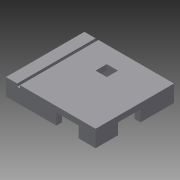
# Autodesk Inventor part: Casing Top
Saved by Autodesk Inventor 2014 SP1 (Build 180222100, 222)
## iProperties
Created: 2013-10-01
Part Number: Casing Top
Material: Generic
Document SubType Name: Modeling
Designer: Anthony
Density: 1 g/cm^3
Appearance: Default
Author: Anthony
Autodesk Inventor part; units mm, degrees
ref_plane "YZ Plane" through (0, 0, 0) normal (1, 0, 0) x (0, 1, 0)
ref_plane "XZ Plane" through (0, 0, 0) normal (0, 1, 0) x (-1, 0, 0)
ref_plane "XY Plane" through (0, 0, 0) normal (0, 0, 1) x (1, 0, 0)
sketch "Sketch1" plane through (0, 0, 0) normal (0, 1, 0) x (-1, 0, 0)
  line L0 (0, 0) -> (-50.8, 0)
  line L1 (-50.8, 0) -> (-50.8, 44.45)
  line L2 (-50.8, 44.45) -> (0, 44.45)
  line L3 (0, 44.45) -> (0, 0)
  dimension "d0" = 50.8
  dimension "d1" = 44.45
  constraints: 8 end point, 2 parallel, 1 horizontal, 1 perpendicular
  measures "d0" distance of L1.end L2.end
  measures "d1" distance of L0.end L1.end
extrude "Extrusion1" add sketch "Sketch1" along normal blind 3.175
sketch "Sketch2" plane through (0, 0, 44.45) normal (0, -1, 0) x (1, 0, 0)
  line L0 (50.8, 0) -> (0, 0)
  line L1 (0, 0) -> (0, -44.45)
  line L2 (0, -44.45) -> (50.8, -44.45)
  line L3 (50.8, -44.45) -> (50.8, 0)
  line L4 (3.175, -3.175) -> (47.625, -3.175)
  line L5 (47.625, -3.175) -> (47.625, -41.275)
  line L6 (47.625, -41.275) -> (3.175, -41.275)
  line L7 (3.175, -41.275) -> (3.175, -3.175)
  dimension "d4" = 3.175
  dimension "d7" = 3.175
  dimension "d5" = 3.175
  dimension "d6" = 3.175
  constraints: 16 end point, 2 parallel, 1 horizontal, 1 perpendicular
  measures "d4" distance between parallel lines of L1 L7
  measures "d7" distance between parallel lines of L0 L4
  measures "d5" distance between parallel lines of L2 L6
  measures "d6" distance between parallel lines of L3 L5
extrude "Extrusion2" add sketch "Sketch2" along normal blind 6.35
sketch "Sketch3" plane through (0, -6.35, 44.45) normal (0, 0, 1) x (1, 0, 0)
  line L0 (28.575, 0) -> (41.275, 0)
  line L1 (41.275, 0) -> (41.275, 6.35)
  line L2 (41.275, 6.35) -> (28.575, 6.35)
  line L3 (28.575, 6.35) -> (28.575, 0)
  line L4 (50.8, 0) -> (0, 0) projected
  line L5 (0, 9.525) -> (50.8, 9.525) projected
  line L6 (0, 9.525) -> (0, 0) projected
  dimension "d18" = 0
  dimension "d20" = 28.575
  dimension "d21" = 41.275
  dimension "d27" = 6.35
  constraints: 8 end point, 2 parallel, 1 horizontal, 1 perpendicular
  measures "d18" distance between parallel lines of L0 L4
  measures "d20" distance between parallel lines of L3 L6
  measures "d21" distance between parallel lines of L6 L1
  measures "d27" distance of L0.end L1.end
extrude "Extrusion3" cut sketch "Sketch3" against normal blind 3.175
sketch "Sketch4" plane through (50.8, 3.175, 44.45) normal (1, 0, 0) x (0, 0, -1)
  line L0 (0, 0) -> (0, -9.525) projected
  line L1 (44.45, -9.525) -> (0, -9.525) projected
  line L2 (12.7, -9.525) -> (25.4, -9.525)
  line L3 (25.4, -9.525) -> (25.4, -3.175)
  line L4 (25.4, -3.175) -> (12.7, -3.175)
  line L5 (12.7, -3.175) -> (12.7, -9.525)
  point P0 (44.45, -3.175)
  dimension "d22" = 6.35
  dimension "d23" = 12.7
  dimension "d24" = 25.4
  constraints: 8 end point, 2 parallel, 1 horizontal, 1 perpendicular, 1 point on line
  measures "d22" distance of L4.end L2.start
  measures "d23" distance between parallel lines of L0 L5
  measures "d24" distance between parallel lines of L0 L3
extrude "Extrusion4" cut sketch "Sketch4" against normal blind 3.175
sketch "Sketch5" plane through (0, 3.175, 0) normal (0, 1, 0) x (1, 0, 0)
  line L0 (50.8, 0) -> (0, 0) projected
  line L1 (0, 0) -> (0, -44.45) projected
  line L2 (22.225, -9.525) -> (28.575, -9.525)
  line L3 (28.575, -9.525) -> (28.575, -15.875)
  line L4 (28.575, -15.875) -> (22.225, -15.875)
  line L5 (22.225, -15.875) -> (22.225, -9.525)
  dimension "d28" = 22.225
  dimension "d29" = 28.575
  dimension "d30" = 9.525
  dimension "d31" = 15.875
  constraints: 8 end point, 2 parallel, 1 horizontal, 1 perpendicular
  measures "d28" distance between parallel lines of L1 L5
  measures "d29" distance between parallel lines of L1 L3
  measures "d30" distance between parallel lines of L0 L2
  measures "d31" distance between parallel lines of L0 L4
extrude "Extrusion5" cut sketch "Sketch5" against normal blind 3.175
sketch "Sketch6" plane through (0, 3.175, 0) normal (0, 1, 0) x (1, 0, 0)
  line L0 (50.8, 0) -> (0, 0) projected
  line L1 (0, 0) -> (0, -44.45) projected
  line L2 (0, -44.45) -> (50.8, -44.45) projected
  line L3 (6.35, 0) -> (7.9375, 0)
  line L4 (7.9375, 0) -> (7.9375, -44.45)
  line L5 (7.9375, -44.45) -> (6.35, -44.45)
  line L6 (6.35, -44.45) -> (6.35, 0)
  dimension "d34" = 1.5875
  dimension "d35" = 6.35
  constraints: 8 end point, 2 parallel, 2 point on line, 1 horizontal, 1 perpendicular
  measures "d34" distance of L3.start L3.end
  measures "d35" distance between parallel lines of L1 L6
extrude "Extrusion6" cut sketch "Sketch6" against normal blind 1.5875 contours L4 L2 L6 L0
body "Solid1"
